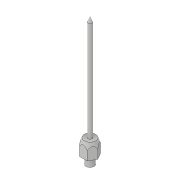
# Autodesk Inventor part: CH_01_0003_injector
Saved by Autodesk Inventor 2019 (Build 230136000, 136)
## iProperties
Created: 2022-02-10
Part Number: CH_01_0003_injector
Material: Generic
Document SubType Name: Modeling
Designer: Tomasz Krakowski
Density: 1 g/cm^3
Appearance: Default
Author: Tomasz Krakowski
Autodesk Inventor part; units mm, degrees
ref_plane "YZ Plane" through (0, 0, 0) normal (1, 0, 0) x (0, 1, 0)
ref_plane "XZ Plane" through (0, 0, 0) normal (0, 1, 0) x (-1, 0, 0)
ref_plane "XY Plane" through (0, 0, 0) normal (0, 0, 1) x (1, 0, 0)
sketch "Sketch1" plane through (0, 0, 0) normal (0, 1, 0) x (-1, 0, 0)
  circle A0 centre (0, 0) radius 1.5
  dimension "d0" = 3
  constraints: 1 centre point, 1 coincident
  measures "d0" diameter of A0
extrude "Extrusion1" add sketch "Sketch1" along normal blind 78
chamfer "Chamfer1" distance 1.5 distance2 4 1 edges at (1.5, 78, 0) measured on face at (1, 78, 0)
sketch "Sketch2" plane through (0, 0, 0) normal (0, -1, 0) x (1, 0, 0)
  circle A0 centre (0, 0) radius 1.5 projected
  line L0 (2.8868, -5) -> (-2.8868, -5)
  line L1 (-2.8868, -5) -> (-5.7735, 0)
  line L2 (-5.7735, 0) -> (-2.8868, 5)
  line L3 (-2.8868, 5) -> (2.8868, 5)
  line L4 (2.8868, 5) -> (5.7735, 0)
  line L5 (5.7735, 0) -> (2.8868, -5)
  dimension "d6" = 10
  constraints: 12 end point, 1 coincident, 1 horizontal, 13 other
  measures "d6" distance between parallel lines of L0 L3
extrude "Extrusion2" add sketch "Sketch2" along normal blind 11 contours A0 | L0 L1 L2 L3 L4 L5
sketch "Sketch3" plane through (0, -11, 0) normal (0, -1, 0) x (1, 0, 0)
  circle A0 centre (0, 0) radius 3
  dimension "d12" = 6
  constraints: 1 centre point, 1 coincident
  measures "d12" diameter of A0
extrude "Extrusion3" add sketch "Sketch3" along normal blind 6
ref_plane "Work Plane1" through (0, -10, 0) normal (0.8660254, 0, 0.5) x (0, 1, 0)
sketch "Sketch5" plane through (0, -10, 0) normal (0.8660254, 0, 0.5) x (0, 1, 0)
  line L0 (10, 4.25) -> (5.5, 5.7735)
  line L1 (10, 5.7735) -> (10, 2.8868) construction
  line L2 (10, 5.7735) -> (-1, 5.7735) construction
  line L3 (-1, 2.8868) -> (-1, 5.7735) construction
  line L4 (10, 2.8868) -> (-1, 2.8868) construction
  line L5 (10, 4.25) -> (10, 5.7735)
  line L6 (5.5, 5.7735) -> (10, 5.7735)
  line L7 (-18.8, 0) -> (105.8, 0) projected
  point P0 (10, 0)
  dimension "d17" = 4.25
  dimension "d18" = 4.5
  constraints: 6 end point, 1 collinear, 1 vertical
  measures "d17" distance of L0.start point (10, 0)
  measures "d18" distance from line of L1 L0.end
revolve "Revolution1" cut sketch "Sketch5" angle 360 about axis through (0, -10, 0) along (0, 1, 0)
body "Solid1"
